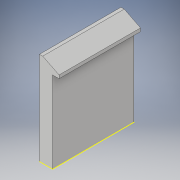
# Autodesk Inventor part: straight2
Saved by Autodesk Inventor 2019 (Build 230136000, 136)
## iProperties
Created: 2019-01-19
Part Number: straight2
Material: Generic
Document SubType Name: Modeling
Designer: assman
Density: 1 g/cm^3
Appearance: Default
Author: assman
Autodesk Inventor part; units mm, degrees
ref_plane "YZ Plane" through (0, 0, 0) normal (1, 0, 0) x (0, 1, 0)
ref_plane "XZ Plane" through (0, 0, 0) normal (0, 1, 0) x (-1, 0, 0)
ref_plane "XY Plane" through (0, 0, 0) normal (0, 0, 1) x (1, 0, 0)
sketch "Sketch1" plane through (0, 0, 0) normal (0, 0, 1) x (1, 0, 0)
  line L0 (-0.8, 0) -> (0.8, 0)
  line L1 (0.8, 0) -> (0.8, 10)
  line L2 (0.8, 10) -> (1.6, 10)
  line L3 (1.6, 10) -> (1.6, 10.4)
  line L4 (1.6, 10.4) -> (-0.4, 11.3967)
  line L5 (-0.4, 11.3967) -> (-0.8, 11.3967)
  line L6 (-0.8, 11.3967) -> (-0.8, 0)
  point P0 (0, 0)
  point P1 (0, 0)
  point P2 (0, 0)
  dimension "width" = 1.6
  dimension "height" = 10
  dimension "d2" = 0.4
  dimension "fixer" = 0.8
  dimension "d4" = 0.4
  constraints: 14 end point, 4 perpendicular, 2 coincident, 1 horizontal, 1 midpoint, 1 parallel
  measures "width" distance of L0.start L0.end
  measures "height" distance of L0.end L1.end
  measures "d2" distance of L2.end L3.end
  measures "fixer" distance of L1.end L2.end
  measures "d4" distance of L4.end L5.end
extrude "Extrusion1" add sketch "Sketch1" along normal blind 10
sketch "Sketch2" plane through (-0.8, 0, 0) normal (0, -1, 0) x (1, 0, 0)
  line L0 (0, 0) -> (1.6, 0) projected
  line L1 (1.6, 0) -> (1.6, 10) projected
  line L2 (0, 10) -> (1.6, 10) projected
  line L3 (0, 0) -> (0, 10) projected
  point P0 (0.8, 0)
  point P1 (0.8, 5)
body "Solid1"
